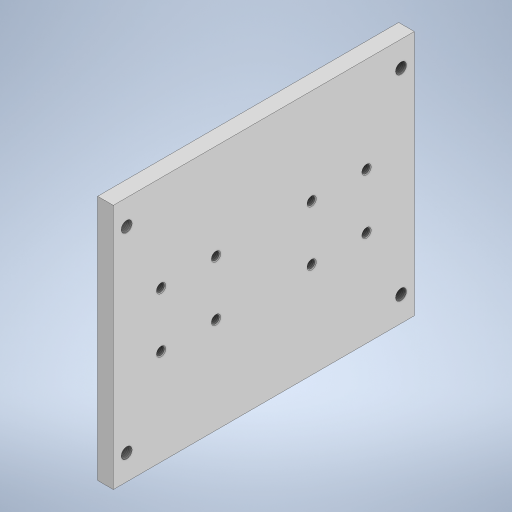
# Autodesk Inventor part: Adapterplatte1Gong_2025-03-28v00r00grm
Saved by Autodesk Inventor 2023.5 (Build 275446000, 446)
## iProperties
Created: 2025-03-27
Part Number: Adapterplatte1Gong_2025-03-28v00r00grm
Material: Generisch
Document SubType Name: Modeling
Designer: student
Density: 1 g/cm^3
Appearance: Vorgabe
Author: student
Autodesk Inventor part; units mm, degrees
ref_plane "YZ Plane" through (0, 0, 0) normal (1, 0, 0) x (0, 1, 0)
ref_plane "XZ Plane" through (0, 0, 0) normal (0, 1, 0) x (-1, 0, 0)
ref_plane "XY Plane" through (0, 0, 0) normal (0, 0, 1) x (1, 0, 0)
sketch "Skizze1" plane through (0, 0, 0) normal (1, 0, 0) x (0, 1, 0)
  line L0 (78.5, 96) -> (-78.5, 96)
  line L1 (-78.5, 96) -> (-78.5, -96)
  line L2 (-78.5, -96) -> (78.5, -96)
  line L3 (78.5, -96) -> (78.5, 96)
  point P0 (0, 0)
  dimension "d0" = 192
  dimension "d1" = 157
  dimension "d2" = 78.5
  dimension "d3" = 96
  constraints: 8 end point, 2 parallel, 1 horizontal, 1 perpendicular
  measures "d0" distance of L2.end L0.start
  measures "d1" distance of L1.end L2.end
  measures "d2" distance from line of point (0, 0) L3
  measures "d3" distance from line of point (0, 0) L2
extrude "Extrusion1" add sketch "Skizze1" along normal blind 10
sketch "草图5" plane through (0, 0, 0) normal (-1, 0, 0) x (0, 0, 1)
  point P0 (0, 0)
sketch "草图6" plane through (10, 0, 0) normal (1, 0, 0) x (0, 0, -1)
  line L0 (-24, 25) -> (-72, 25)
  line L1 (-72, 25) -> (-72, -25)
  line L2 (-72, -25) -> (-24, -25)
  line L3 (-24, -25) -> (-24, 25)
  line L4 (-24, 25) -> (-72, -25) construction
  line L5 (-72, 25) -> (-24, -25) construction
  line L6 (-96, 78.5) -> (-96, -78.5) projected
  line L7 (-65.5, -17.5) -> (-30.5, -17.5)
  line L8 (-30.5, -17.5) -> (-30.5, 17.5)
  line L9 (-30.5, 17.5) -> (-65.5, 17.5)
  line L10 (-65.5, 17.5) -> (-65.5, -17.5)
  line L11 (-65.5, -17.5) -> (-30.5, 17.5) construction
  line L12 (-30.5, -17.5) -> (-65.5, 17.5) construction
  circle A0 centre (-65.5, -17.5) radius 2.5
  circle A1 centre (-30.5, -17.5) radius 2.5
  circle A2 centre (-30.5, 17.5) radius 2.5
  circle A3 centre (-65.5, 17.5) radius 2.5
  line L13 (24, 25) -> (72, 25)
  line L14 (72, 25) -> (72, -25)
  line L15 (72, -25) -> (24, -25)
  line L16 (24, -25) -> (24, 25)
  line L17 (24, 25) -> (72, -25) construction
  line L18 (72, 25) -> (24, -25) construction
  line L19 (65.5, -17.5) -> (30.5, -17.5)
  line L20 (30.5, -17.5) -> (30.5, 17.5)
  line L21 (30.5, 17.5) -> (65.5, 17.5)
  line L22 (65.5, 17.5) -> (65.5, -17.5)
  line L23 (65.5, -17.5) -> (30.5, 17.5) construction
  line L24 (30.5, -17.5) -> (65.5, 17.5) construction
  circle A4 centre (65.5, -17.5) radius 2.5
  circle A5 centre (30.5, -17.5) radius 2.5
  circle A6 centre (30.5, 17.5) radius 2.5
  circle A7 centre (65.5, 17.5) radius 2.5
  point P0 (0, 0)
  point P1 (-48, 0)
  point P2 (-48, 0)
  point P3 (48, 0)
  point P4 (48, 0)
  dimension "d31" = 50
  dimension "d32" = 48
  dimension "d33" = 24
  dimension "d34" = 35
  dimension "d35" = 35
  dimension "d36" = 5
  dimension "d39" = 360
  dimension "d48" = 5
  dimension "d49" = 5
  dimension "d50" = 5
  dimension "d51" = 5
  constraints: 48 end point, 8 centre point, 4 coincident, 4 midpoint, 4 parallel, 2 horizontal, 2 perpendicular, 9 other
  measures "d31" distance of L0.end L1.end
  measures "d32" distance of L0.start L0.end
  measures "d33" distance between parallel lines of L1 L6
  measures "d34" distance of L9.end L7.start
  measures "d35" distance of L7.start L7.end
  measures "d36" diameter of A0
  measures "d48" diameter of A6
  measures "d49" diameter of A5
  measures "d50" diameter of A7
  measures "d51" diameter of A4
hole "孔1" at (10, -17.5, 65.5) at (10, 17.5, 65.5) at (10, -17.5, 30.5) at (10, -17.5, -30.5) at (10, 17.5, -30.5) at (10, 17.5, -65.5) at (10, -17.5, -65.5) at (10, 17.5, 65.5) at (10, 17.5, 30.5) direction (-1, 0, 0) diameter 4.917 end through all thread size "M6x1" class "6H" standard "ISO Metric profile"
chamfer "倒角1" distance 0.5 angle 45 8 edges at (10, -17.5, -63.0415) (10, -17.5, -28.0415) (10, 17.5, -63.0415) (10, 17.5, -28.0415) (10, -17.5, 32.9585) (10, -17.5, 67.9585) (10, 17.5, 32.9585) (10, 17.5, 67.9585)
sketch "草图10" plane through (10, 0, 0) normal (1, 0, 0) x (0, 0, -1)
  line L0 (-169, 0) -> (145, 0)
  line L1 (0, 114) -> (0, -130)
  line L2 (-96, 78.5) -> (-96, -78.5) projected
  line L3 (-87.5, 62.5) -> (87.5, 62.5)
  line L4 (87.5, 62.5) -> (87.5, -62.5)
  line L5 (87.5, -62.5) -> (-87.5, -62.5)
  line L6 (-87.5, -62.5) -> (-87.5, 62.5)
  line L7 (-87.5, 62.5) -> (87.5, -62.5) construction
  line L8 (87.5, 62.5) -> (-87.5, -62.5) construction
  circle A0 centre (-87.5, 62.5) radius 3.25
  circle A1 centre (-87.5, -62.5) radius 3.25
  circle A2 centre (87.5, 62.5) radius 3.25
  circle A3 centre (87.5, -62.5) radius 3.25
  point P0 (0, 0)
  dimension "d74" = 96
  dimension "d75" = 175
  dimension "d76" = 125
  dimension "d77" = 6.5
  constraints: 16 end point, 4 centre point, 3 symmetric about line, 2 horizontal, 2 midpoint, 2 parallel, 1 coincident, 1 perpendicular, 1 vertical, 3 other
  measures "d74" distance between parallel lines of L2 L1
  measures "d75" distance of L3.start L3.end
  measures "d76" distance of L3.end L4.end
  measures "d77" diameter of A0
extrude "拉伸5" cut sketch "草图10" against normal blind 10 contours A1 L5 L6 | L6 L5 A1 | A0 L3 L6 | L6 L3 A0 | A2 L3 L4 | L4 L3 A2 | A3 L5 L4 | L4 L5 A3
thread "螺纹6" size "M7x1" class "6H" standard "ANSI Metric M Profile" length 10
thread "螺纹7" size "M7x1" class "6H" standard "ANSI Metric M Profile" length 10
thread "螺纹8" size "M7x1" class "6H" standard "ANSI Metric M Profile" length 10
thread "螺纹9" size "M7x1" class "6H" standard "ANSI Metric M Profile" length 10
chamfer "倒角4" distance 0.2 angle 45 4 edges at (10, -62.5, 90.75) (10, -62.5, -84.25) (10, 62.5, -84.25) (10, 62.5, 90.75)
